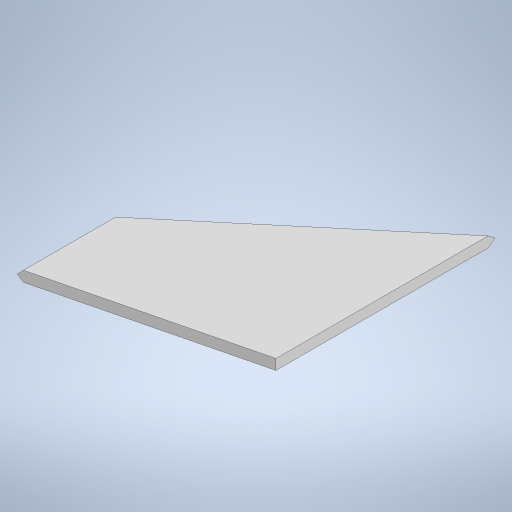
# Autodesk Inventor part: 날개1
Saved by Autodesk Inventor 2023 (Build 270158000, 158)
## iProperties
Created: 2023-08-28
Part Number: 날개1
Material: 일반
Document SubType Name: Modeling
Designer: rlatk
Density: 1 g/cm^3
Appearance: 기본값
Author: rlatk
Autodesk Inventor part; units mm, degrees
ref_plane "YZ Plane" through (0, 0, 0) normal (1, 0, 0) x (0, 1, 0)
ref_plane "XZ Plane" through (0, 0, 0) normal (0, 1, 0) x (-1, 0, 0)
ref_plane "XY Plane" through (0, 0, 0) normal (0, 0, 1) x (1, 0, 0)
sketch "스케치1" plane through (0, 0, 0) normal (0, 1, 0) x (-1, 0, 0)
  line L0 (0, 0) -> (100, 0)
  line L1 (100, 0) -> (100, -130)
  line L2 (100, -130) -> (0, -130)
  line L3 (0, -130) -> (0, 0)
  line L4 (0, -130) -> (92.3211, -52.5334)
  line L5 (0, -130) -> (120.5166, -130) construction
  line L6 (92.3211, -52.5334) -> (100, -46.09)
  line L7 (100, 0) -> (0, -24.6121)
  dimension "d0" = 100
  dimension "d1" = 130
  dimension "d2" = 40
  constraints: 16 end point, 3 point on line, 2 horizontal, 2 parallel, 1 equal length, 1 perpendicular
  measures "d0" distance of L1.end L2.end
  measures "d1" distance of L0.end L1.end
  measures "d2" angle of L5 L4
extrude "돌출1" add sketch "스케치1" along normal blind 5 contours L1 L6 L4 L3 L7
chamfer "모따기1" distance 2.5 angle 45 4 edges at (-46.1605, 5, -91.2667) (-46.1605, 0, -91.2667) (-100, 5, -23.045) (-100, 0, -23.045)
